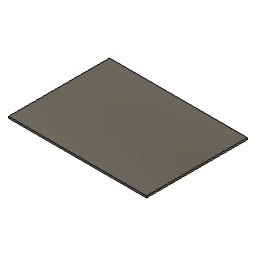
Floor  3 v4 (Autodesk Fusion 360 design; units mm, degrees)
Autodesk Fusion 360 part; units mm, degrees
sketch "Sketch1" plane through (0, 0, 0) normal (0, 0, 1) x (1, 0, 0)
  line L0 (-205, 150) -> (205, 150)
  line L1 (205, 150) -> (205, -150)
  line L2 (205, -150) -> (-205, -150)
  line L3 (-205, -150) -> (-205, 150)
  line L4 (-205, 150) -> (205, -150) construction
  dimension "d1" = 410
  dimension "d2" = 300
  constraint horizontal L0
  constraint vertical L1
  constraint horizontal L2
  constraint vertical L3
  constraint midpoint origin L4
  measures "d1" distance of L0.start L0.end
  measures "d2" distance of L0.start L2.end
extrude "Extrude1" add sketch "Sketch1" along normal blind 5
